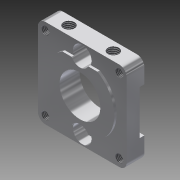
# Autodesk Inventor part: P60 Gearbox End Plate 2
Saved by Autodesk Inventor 2014 SP1 (Build 180222100, 222)
## iProperties
Created: 2012-01-14
Part Number: P60 Gearbox End Plate 2
Material: Aluminum 6061
Document SubType Name: Modeling
Designer: Moses
Density: 2.71 g/cm^3
Mass: 19.722 g
Surface Area: 51.5724 cm^2
Volume: 7.2775 cm^3
Appearance: Aluminum - Polished
Author: Moses
Autodesk Inventor part; units mm, degrees
note: some values were not read from the file. Chosen so that the rebuilt part matches the saved one: sketch regions of "Extrusion1".
ref_plane "YZ Plane" through (0, 0, 0) normal (1, 0, 0) x (0, 1, 0)
ref_plane "XZ Plane" through (0, 0, 0) normal (0, 1, 0) x (-1, 0, 0)
ref_plane "XY Plane" through (0, 0, 0) normal (0, 0, 1) x (1, 0, 0)
sketch "Sketch1" plane through (0, 0, 0) normal (0, 0, 1) x (1, 0, 0)
  line L0 (0, 0) -> (38.1, 0)
  line L1 (38.1, 0) -> (38.1, 38.1)
  line L2 (38.1, 38.1) -> (0, 38.1)
  line L3 (0, 38.1) -> (0, 0)
  circle A0 centre (3.175, 34.925) radius 1.75
  circle A1 centre (34.925, 34.925) radius 1.75
  circle A2 centre (3.175, 3.175) radius 1.75
  circle A3 centre (34.925, 3.175) radius 1.75
  line L4 (0, 19.05) -> (19.05, 19.05)
  circle A4 centre (19.05, 19.05) radius 8.75
  circle A5 centre (19.05, 19.05) radius 6.35
  line L5 (6.83, 34.925) -> (6.83, 38.1)
  line L6 (0, 31.27) -> (3.175, 31.27)
  arc A6 (3.175, 31.27) -> (6.83, 34.925) centre (3.175, 34.925) ccw
  line L7 (4.925, 34.925) -> (6.83, 34.925)
  line L8 (3.175, 6.83) -> (0, 6.83)
  line L9 (6.83, 0) -> (6.83, 3.175)
  arc A7 (6.83, 3.175) -> (3.175, 6.83) centre (3.175, 3.175) ccw
  line L10 (31.27, 3.175) -> (31.27, 0)
  line L11 (38.1, 6.83) -> (34.925, 6.83)
  arc A8 (34.925, 6.83) -> (31.27, 3.175) centre (34.925, 3.175) ccw
  line L12 (34.925, 31.27) -> (38.1, 31.27)
  line L13 (31.27, 38.1) -> (31.27, 34.925)
  arc A9 (31.27, 34.925) -> (34.925, 31.27) centre (34.925, 34.925) ccw
  line L14 (0, 6.83) -> (0, 0)
  line L15 (0, 0) -> (6.83, 0)
  line L16 (31.27, 0) -> (38.1, 0)
  line L17 (38.1, 0) -> (38.1, 6.83)
  line L18 (31.27, 38.1) -> (38.1, 38.1)
  line L19 (38.1, 38.1) -> (38.1, 31.27)
  dimension "d2" = 3.5
  dimension "d0" = 38.1
  dimension "d1" = 38.1
  dimension "d5" = 31.75
  dimension "d8" = 31.75
  dimension "d11" = 3.175
  dimension "d12" = 3.175
  dimension "d13" = 19.05
  dimension "d14" = 17.5
  dimension "d15" = 12.7
  dimension "d16" = 3.175
  dimension "d17" = 3.175
  dimension "d18" = 1.905
  dimension "d24" = 360
  constraints: 40 end point, 9 centre point, 8 point on circle, 5 perpendicular, 3 coincident, 2 horizontal, 2 parallel, 2 point on line, 1 collinear, 1 horizontal alignment, 1 midpoint, 1 vertical, 41 other
  measures "d0" distance of L0.start L0.end
  measures "d1" distance of L0.end L1.end
  measures "d5" distance of point (3.175, 34.925) A1.centre
  measures "d8" distance of point (3.175, 34.925) A2.centre
  measures "d11" distance from line of L2 point (3.175, 34.925)
  measures "d12" distance from line of L3 point (3.175, 34.925)
  measures "d13" distance of L4.start L4.end
  measures "d14" diameter of A4
  measures "d15" diameter of A5
  measures "d16" distance of L5.start L5.end
  measures "d17" distance of L6.start L6.end
  measures "d18" distance of L7.start L5.start
extrude "Extrusion1" add sketch "Sketch1" along normal blind 7.62 contours L3 L8 A7 L9 L0 | L9 A7 L8 L3 L6 A6 L5 L2 L13 A9 L12 L1 L11 A8 L10 L0 | L10 A8 L11 L1 L0 | L3 L2 L5 A6 L6 | L12 A9 L13 L2 L1
fillet "Fillet1" radius 3.175 4 edges at (0, 38.1, 3.81) (38.1, 38.1, 3.81) (0, 0, 3.81) (38.1, 0, 3.81)
sketch "Sketch2" plane through (3.175, 38.1, 0) normal (0, 1, 0) x (1, 0, 0)
  line L0 (31.75, 0) -> (0, 0) projected
  line L1 (0, -7.62) -> (31.75, -7.62) projected
  line L2 (15.875, 0) -> (15.875, -3.81)
  line L3 (15.875, -3.81) -> (25.4, -3.81)
  line L4 (15.875, -3.81) -> (6.35, -3.81)
  circle A0 centre (25.4, -3.81) radius 2.3495
  circle A1 centre (6.35, -3.81) radius 2.3495
  point P0 (-3.175, 0)
  dimension "d29" = 3.81
  dimension "d30" = 9.525
  dimension "d31" = 9.525
  dimension "d32" = 4.699
  dimension "d33" = 4.699
  constraints: 6 end point, 2 centre point, 2 coincident, 2 perpendicular, 1 collinear, 1 midpoint
  measures "d29" distance of L2.start L2.end
  measures "d30" distance of L2.end L3.end
  measures "d31" distance of L2.end L4.end
  measures "d32" diameter of A0
  measures "d33" diameter of A1
extrude "Extrusion2" cut sketch "Sketch2" against normal blind 7.62
sketch "Sketch3" plane through (3.175, 0, 0) normal (0, -1, 0) x (1, 0, 0)
  line L0 (0, 0) -> (31.75, 0) projected
  line L1 (15.875, 0) -> (15.875, 3.81)
  line L2 (15.875, 3.81) -> (6.35, 3.81)
  line L3 (15.875, 3.81) -> (25.4, 3.81)
  circle A0 centre (6.35, 3.81) radius 2.3495
  circle A1 centre (25.4, 3.81) radius 2.3495
  point P0 (-3.175, 0)
  dimension "d36" = 3.81
  dimension "d37" = 9.525
  dimension "d38" = 9.525
  dimension "d39" = 4.699
  dimension "d40" = 4.699
  constraints: 6 end point, 2 centre point, 2 coincident, 2 perpendicular, 1 collinear, 1 midpoint
  measures "d36" distance of L1.start L1.end
  measures "d37" distance of L1.end L2.end
  measures "d38" distance of L1.end L3.end
  measures "d39" diameter of A0
  measures "d40" diameter of A1
extrude "Extrusion3" cut sketch "Sketch3" against normal blind 7.62
thread "Thread1" size "M3.5x0.6" class "6H" standard "ANSI Metric M Profile" full length
thread "Thread2" size "M3.5x0.6" class "6H" standard "ANSI Metric M Profile" full length
thread "Thread3" size "M3.5x0.6" class "6H" standard "ANSI Metric M Profile" full length
thread "Thread4" size "M3.5x0.6" class "6H" standard "ANSI Metric M Profile" full length
thread "Thread5" size "10-32 UNF" class "2B" standard "ANSI Unified Screw Threads" full length
thread "Thread6" size "10-32 UNF" class "2B" standard "ANSI Unified Screw Threads" full length
thread "Thread7" size "10-32 UNF" class "2B" standard "ANSI Unified Screw Threads" full length
thread "Thread8" size "10-32 UNF" class "2B" standard "ANSI Unified Screw Threads" full length
sketch "Sketch4" plane through (0, 0, 0) normal (0, 0, -1) x (-1, 0, 0)
  line L0 (0, 34.925) -> (0, 3.175) projected
  line L1 (-38.1, 3.175) -> (-38.1, 34.925) projected
  circle A0 centre (-19.05, 19.05) radius 8.75 projected
  line L2 (0, 19.05) -> (-38.1, 19.05) construction
  line L3 (-10.3, 9.55) -> (-10.3, 28.55) construction
  line L4 (-27.8, 9.55) -> (-27.8, 28.55) construction
  line L5 (0, 9.55) -> (-15.24, 9.55)
  line L6 (-38.1, 9.55) -> (-22.86, 9.55)
  line L7 (0, 28.55) -> (-15.24, 28.55)
  line L8 (-38.1, 28.55) -> (-22.86, 28.55)
  circle A1 centre (-19.05, 19.05) radius 9.25
  line L9 (-15.24, 9.55) -> (-12.2627, 12.7655)
  line L10 (-15.24, 28.55) -> (-12.2627, 25.3345)
  line L11 (-22.86, 28.55) -> (-25.8373, 25.3345)
  line L12 (-22.86, 9.55) -> (-25.8373, 12.7655)
  point P0 (0, 0)
  point P1 (-10.3, 19.05)
  point P2 (-27.8, 19.05)
  dimension "d59" = 19
  dimension "d60" = 0.5
  dimension "d61" = 15.24
  constraints: 22 end point, 10 point on line, 8 equal length, 6 point on circle, 4 midpoint, 4 tangent, 2 perpendicular, 1 centre point
  measures "d59" distance of L3.start L3.end
  measures "d60" radial gap between concentric circles of A0 A1
  measures "d61" distance of L5.start L5.end
extrude "Extrusion4" cut sketch "Sketch4" against normal blind 2 contours L0 L5 L9 A1 L10 L7 | A1 L12 L6 L1 L8 L11
fillet "Fillet2" radius 3.175 4 edges at (22.86, 9.55, 1) (22.86, 28.55, 1) (15.24, 28.55, 1) (15.24, 9.55, 1)
sketch "Sketch5" plane through (0, 0, 7.62) normal (0, 0, 1) x (1, 0, 0)
  circle A0 centre (19.05, 19.05) radius 8.75 projected
  line L0 (34.925, 0) -> (3.175, 0) projected
  circle A1 centre (19.05, 33.55) radius 4
  circle A2 centre (19.05, 4.55) radius 4
  line L1 (19.05, 33.55) -> (19.05, 4.55) construction
  line L2 (11.55, 31.7509) -> (15.4774, 31.7509)
  line L3 (22.6226, 31.7509) -> (26.55, 31.7509)
  arc A3 (11.55, 31.7509) -> (11.55, 6.3491) centre (19.05, 19.05) ccw
  arc A4 (26.55, 6.3491) -> (26.55, 31.7509) centre (19.05, 19.05) ccw
  line L4 (11.55, 6.3491) -> (15.4774, 6.3491)
  line L5 (22.6226, 6.3491) -> (26.55, 6.3491)
  line L6 (15.4774, 31.7509) -> (22.6226, 31.7509) construction
  line L7 (15.4774, 6.3491) -> (22.6226, 6.3491) construction
  circle A5 centre (19.05, 33.55) radius 2.3495
  circle A6 centre (19.05, 4.55) radius 2.3495
  point P0 (0, 0)
  dimension "d66" = 29
  dimension "d67" = 8
  dimension "d68" = 15
  dimension "d69" = 14.75
  dimension "d72" = 4.699
  constraints: 14 end point, 8 point on circle, 7 parallel, 6 centre point, 4 coincident, 4 perpendicular, 3 equal radius, 1 midpoint
  measures "d66" distance of L1.start L1.end
  measures "d67" diameter of A1
  measures "d68" distance of L3.end L2.start
  measures "d69" radius of A4
  measures "d72" diameter of A5
extrude "Extrusion5" add sketch "Sketch5" along normal blind 1 contours A1 L3 A4 L5 A2 L4 A3 L2
extrude "Extrusion6" cut sketch "Sketch5" against normal blind 7.62 contours A5 | A6
extrude "Extrusion7" cut sketch "Sketch5" against normal blind 5.62 contours A1 | A2
equation "\"d16\" = d11"
equation "\"d17\" = d11"
body "Solid1"
